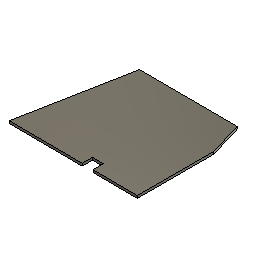
oceaan-25-floor_6 v2 (Autodesk Fusion 360 design; units mm, degrees)
Autodesk Fusion 360 part; units mm, degrees
note: some values were not read from the file. Set by a fixed rule: which sketch regions a step uses.
sketch "Sketch1" plane through (0, 0, 0) normal (0, 1, 0) x (1, 0, 0)
  line L0 (-171, -3.3746) -> (-171, 49.6266)
  line L1 (-227, -2.9929) -> (-227, 50.0083)
  line L2 (-227, 50.0083) -> (-171, 49.6266)
  line L3 (6.2247, 557.2673) -> (-495.7717, 559.1655)
  line L4 (57, 386.8074) -> (57, -4.9287)
  line L5 (57, 386.8074) -> (6.2247, 557.2673)
  line L6 (-495.7717, 559.1655) -> (-602, -0.4369)
  line L7 (57, -4.9287) -> (-171, -3.3746)
  line L8 (-227, -2.9929) -> (-602, -0.4369)
  dimension "d9" = 502
  dimension "d13" = 659
  dimension "d14" = 562
  dimension "d15" = 560
  dimension "d18" = 228
  dimension "d19" = 284
  dimension "d23" = 53
  constraint collinear L7 L8
  constraint parallel L2 L7
  measures "d9" distance of L3.start L3.end
  measures "d13" distance of L6.end L4
  measures "d14" distance of L4.end L3
  measures "d15" distance of L6.end L3
  measures "d18" distance of L4 L0.start
  measures "d19" distance of L4 L1.start
  measures "d23" distance of L2 L7
extrude "Extrude1" add sketch "Sketch1" along normal blind 12.5
equation "d19 = 289.00 mm - 5 mm"
